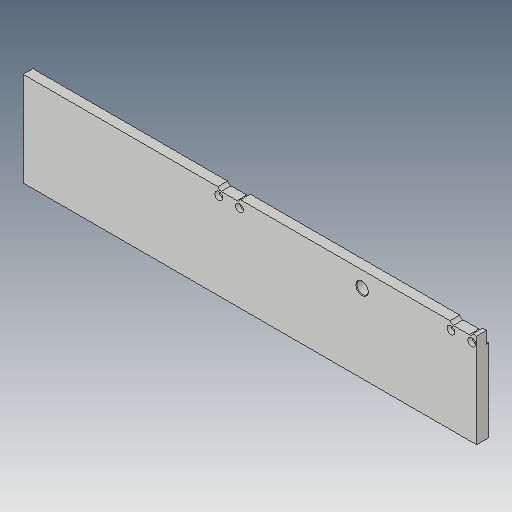
# Autodesk Inventor part: Frame Front
Saved by Autodesk Inventor 2019 (Build 230136000, 136)
## iProperties
Created: 2019-02-26
Part Number: Frame Front
Material: Generic
Document SubType Name: Modeling
Designer: LillaHunden
Density: 1 g/cm^3
Appearance: Default
Author: LillaHunden
Autodesk Inventor part; units mm, degrees
ref_plane "YZ Plane" through (0, 0, 0) normal (1, 0, 0) x (0, 1, 0)
ref_plane "XZ Plane" through (0, 0, 0) normal (0, 1, 0) x (-1, 0, 0)
ref_plane "XY Plane" through (0, 0, 0) normal (0, 0, 1) x (1, 0, 0)
sketch "Sketch1" plane through (0, 0, 0) normal (0, 0, 1) x (1, 0, 0)
  line L0 (-156, 9.9823) -> (3.1716, 9.9823) projected
  line L1 (215, 9.9823) -> (215, -67) projected
  line L2 (215, -67) -> (-156, -67) projected
  line L3 (-156, -67) -> (-156, 9.9823) projected
  circle A0 centre (121.3, -3.0177) radius 5.2625 projected
  arc A1 (193.1716, 9.9823) -> (196, 7.9823) centre (196, 10.9823) ccw projected
  line L4 (196, 7.9823) -> (209, 7.9823) projected
  arc A2 (209, 7.9823) -> (211.8284, 9.9823) centre (209, 10.9823) ccw projected
  line L5 (211.8284, 9.9823) -> (215, 9.9823) projected
  arc A3 (3.1716, 9.9823) -> (6, 7.9823) centre (6, 10.9823) ccw projected
  line L6 (6, 7.9823) -> (19, 7.9823) projected
  arc A4 (19, 7.9823) -> (21.8284, 9.9823) centre (19, 10.9823) ccw projected
  line L7 (21.8284, 9.9823) -> (193.1716, 9.9823) projected
  line L8 (69.5, -23) -> (69.5, -39) projected
  arc A5 (69.5, -39) -> (76.5, -39) centre (73, -39) ccw projected
  line L9 (76.5, -39) -> (76.5, -23) projected
  arc A6 (76.5, -23) -> (69.5, -23) centre (73, -23) ccw projected
  arc A7 (46.83, -62.57) -> (52.03, -62.57) centre (49.43, -62.57) ccw projected
  line L10 (52.03, -62.57) -> (52.03, -46.57) projected
  arc A8 (52.03, -46.57) -> (46.83, -46.57) centre (49.43, -46.57) ccw projected
  line L11 (46.83, -46.57) -> (46.83, -62.57) projected
  arc A9 (46.83, -15.43) -> (52.03, -15.43) centre (49.43, -15.43) ccw projected
  line L12 (52.03, -15.43) -> (52.03, 0.57) projected
  arc A10 (52.03, 0.57) -> (46.83, 0.57) centre (49.43, 0.57) ccw projected
  line L13 (46.83, 0.57) -> (46.83, -15.43) projected
  arc A11 (93.97, -15.43) -> (99.17, -15.43) centre (96.57, -15.43) ccw projected
  line L14 (99.17, -15.43) -> (99.17, 0.57) projected
  arc A12 (99.17, 0.57) -> (93.97, 0.57) centre (96.57, 0.57) ccw projected
  line L15 (93.97, 0.57) -> (93.97, -15.43) projected
  arc A13 (93.97, -62.57) -> (99.17, -62.57) centre (96.57, -62.57) ccw projected
  line L16 (99.17, -62.57) -> (99.17, -46.57) projected
  arc A14 (99.17, -46.57) -> (93.97, -46.57) centre (96.57, -46.57) ccw projected
  line L17 (93.97, -46.57) -> (93.97, -62.57) projected
  circle A15 centre (21, 3.7521) radius 3.25 projected
  circle A16 centre (211, 3.7521) radius 3.25 projected
  circle A17 centre (194, 3.7521) radius 3.25 projected
  circle A18 centre (4, 3.7521) radius 3.25 projected
  circle A19 centre (-123.8333, -6.3333) radius 3.25 projected
  circle A20 centre (-123.8333, -14.3333) radius 3.25 projected
  circle A21 centre (26.1667, -14.3333) radius 3.25 projected
  circle A22 centre (-3.8333, -14.3333) radius 3.25 projected
  circle A23 centre (-33.8333, -6.3333) radius 3.25 projected
  circle A24 centre (-63.8333, -14.3333) radius 3.25 projected
  circle A25 centre (-93.8333, -14.3333) radius 3.25 projected
  circle A26 centre (-93.8333, -6.3333) radius 3.25 projected
  circle A27 centre (-63.8333, -6.3333) radius 3.25 projected
  circle A28 centre (-33.8333, -14.3333) radius 3.25 projected
  circle A29 centre (-3.8333, -6.3333) radius 3.25 projected
  circle A30 centre (26.1667, -6.3333) radius 3.25 projected
  point P0 (0, 0)
extrude "Extrusion1" add sketch "Sketch1" along normal blind 10 contours L0 A3 L6 A4 L7 A1 L4 A2 L5 L1 L2 L3 | A0 | A6 L9 A5 L8 | L11 A8 L10 A7 | L13 A10 L12 A9 | L15 A12 L14 A11 | L17 A14 L16 A13 | A15 | A16 | A17 | A18 | A19 | A20 | A21 | A22 | A23 | A24 | A25 | A26 | A27 | A28 | A29 | A30
sketch "Sketch2" plane through (215, -67, 0) normal (1, 0, 0) x (0, 0, -1)
  line L0 (282, 67) -> (-2, 67) construction
  line L1 (282, 67) -> (282, 76.9823) construction
  line L2 (-2, 76.9823) -> (282, 76.9823) construction
  line L3 (0, 0) -> (0, 76.9823) construction
  line L4 (0, 76.9823) -> (-10, 76.9823) construction
  line L5 (-10, 0) -> (-10, 76.9823) construction
  line L6 (0, 0) -> (-10, 0) construction
  line L7 (0, 76.9823) -> (0, 0) projected
  line L8 (0, 76.9823) -> (-2, 76.9823)
  line L9 (-2, 76.9823) -> (-2, 67)
  line L10 (-2, 67) -> (0, 67)
  line L11 (0, 67) -> (0, 76.9823)
  line L12 (-2, 76.9823) -> (-2, 67) projected
  point P0 (0, 67)
  constraints: 8 end point, 2 parallel, 1 horizontal, 1 perpendicular
extrude "Extrusion2" cut sketch "Sketch2" against normal through all
sketch "Sketch3" plane through (0, 0, 0) normal (0, 0, -1) x (-1, 0, 0)
  point P0 (0, 0)
sketch "Sketch4" plane through (0, 0, 0) normal (0, 0, -1) x (-1, 0, 0)
  circle A0 centre (-121.3, -3.0177) radius 2.5 construction
  arc A1 (-127.7, -10.7014) -> (-114.9, -10.7014) centre (-121.3, -3.0177) ccw
  arc A2 (-127.7, -10.7014) -> (-157.269, 0) centre (-157.269, -46.2018) ccw
  line L0 (156, 0) -> (-215, 0) projected
  line L1 (-121.3, -3.0177) -> (-121.3, 6.9823) construction
  line L2 (-3.1716, 9.9823) -> (156, 9.9823) projected
  arc A3 (-85.331, 0) -> (-114.9, -10.7014) centre (-85.331, -46.2018) ccw
  line L3 (-157.269, 0) -> (-85.331, 0)
  point P0 (0, 0)
  point P1 (-215, 9.9823)
  point P2 (-193.1716, 9.9823)
  dimension "d4" = 20
  constraints: 6 point on circle, 4 centre point, 4 end point, 3 symmetric about line, 3 tangent, 1 coincident, 1 collinear, 1 perpendicular, 1 point on line, 1 other
  measures "d4" diameter of A1
extrude "Extrusion3" cut sketch "Sketch4" against normal up to surface (2 mm away)
sketch "Sketch5" plane through (215, 0, 2) normal (0, 0, -1) x (-1, 0, 0)
  circle A0 centre (93.7, -3.0177) radius 4.7625 construction
  circle A1 centre (93.7, -3.0177) radius 4.7125
  point P0 (215, 0)
  dimension "d7" = 0.05
  constraints: 1 centre point
  measures "d7" radial gap between concentric circles of A0 A1
extrude "Extrusion4" cut sketch "Sketch5" against normal through all
chamfer "Chamfer1" distance 0.5 angle 45 1 edges at (126.0125, -3.0177, 10)
chamfer "Chamfer2" distance 0.5 angle 45 1 edges at (126.0125, -3.0177, 2)
sketch "Sketch6" plane through (0, 0, 10) normal (0, 0, 1) x (1, 0, 0)
  circle A0 centre (211, 3.7521) radius 1.7 projected
  circle A1 centre (194, 3.7521) radius 1.7 projected
  circle A2 centre (4, 3.7521) radius 1.7 projected
  circle A3 centre (21, 3.7521) radius 1.7 projected
  point P0 (0, 0)
hole "Hole1" at (211, 3.7521, 10) at (194, 3.7521, 10) at (21, 3.7521, 10) at (4, 3.7521, 10) direction (0, 0, -1) diameter 3.4 depth 14.2 counterbore diameter 6.5 counterbore depth 3.4 clearance for "Socket Head Cap Screw ISO 4762" size "M3" standard "ISO"
body "Solid1"
